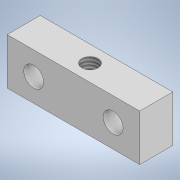
# Autodesk Inventor part: シリンダーの先に着けるやつ
Saved by Autodesk Inventor 2022 (Build 260153070, 153G)
## iProperties
Created: 2022-09-26
Part Number: シリンダーの先に着けるやつ
Material: 一般
Document SubType Name: Modeling
Designer: hirok
Density: 1 g/cm^3
Appearance: 既定
Author: hirok
Autodesk Inventor part; units mm, degrees
ref_plane "YZ Plane" through (0, 0, 0) normal (1, 0, 0) x (0, 1, 0)
ref_plane "XZ Plane" through (0, 0, 0) normal (0, 1, 0) x (-1, 0, 0)
ref_plane "XY Plane" through (0, 0, 0) normal (0, 0, 1) x (1, 0, 0)
sketch "スケッチ1" plane through (0, 0, 0) normal (0, 0, 1) x (1, 0, 0)
  line L0 (0, 0) -> (20, 0)
  line L1 (20, 0) -> (20, 7)
  line L2 (20, 7) -> (0, 7)
  line L3 (0, 7) -> (0, 0)
  dimension "d0" = 7
  dimension "d1" = 20
  constraints: 8 end point, 2 parallel, 1 horizontal, 1 perpendicular
  measures "d0" distance of L0.end L1.end
  measures "d1" distance of L1.end L2.end
extrude "押し出し1" add sketch "スケッチ1" along normal blind 5
sketch "スケッチ2" plane through (0, 7, 0) normal (0, 1, 0) x (1, 0, 0)
  line L0 (20, 0) -> (0, 0) projected
  point P0 (10, -2.5)
  dimension "d4" = 2.5
  measures "d4" distance from line of L0 point (10, -2.5)
hole "穴1" at (10, 7, 2.5) direction (0, -1, 0) diameter 2.459 end through all thread size "M3x0.5" class "6H" standard "ISO Metric profile"
sketch "スケッチ3" plane through (0, 0, 5) normal (0, 0, 1) x (1, 0, 0)
  line L0 (8.7705, 7) -> (11.2295, 7) projected
  line L1 (10, 7) -> (10, 0)
  line L2 (20, 7) -> (0, 7) projected
  point P0 (0, 0)
  point P1 (4, 3.5)
  point P2 (16, 3.5)
  dimension "d12" = 6
  dimension "d13" = 3.5
  constraints: 2 end point, 1 midpoint, 1 symmetric about line, 1 vertical
  measures "d12" distance from line of L1 point (4, 3.5)
  measures "d13" distance from line of L2 point (4, 3.5)
hole "穴2" at (4, 3.5, 5) at (16, 3.5, 5) direction (0, 0, -1) diameter 3 depth 20 tip angle 118
